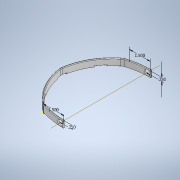
# Autodesk Inventor part: FaceMask_Part1
Saved by Autodesk Inventor 2020 (Build 240168000, 168)
## iProperties
Created: 2020-04-12
Part Number: FaceMask_Part1
Material: Generic
Document SubType Name: Modeling
Designer: maple
Density: 1 g/cm^3
Appearance: Default
Author: maple
Autodesk Inventor part; units mm, degrees
ref_plane "YZ Plane" through (0, 0, 0) normal (1, 0, 0) x (0, 1, 0)
sketch "Sketch1" plane through (0, 0, 0) normal (0, 1, 0) x (-1, 0, 0)
  line L0 (0, 0) -> (-76.2, 0)
  line L1 (-76.2, 0) -> (-76.2, -147.32)
  line L2 (-76.2, -147.32) -> (0, -147.32)
  line L3 (0, -147.32) -> (0, 0)
  line L4 (0, -73.66) -> (0, -139.7)
  line L5 (0, -73.66) -> (0, -7.62)
  line L6 (0, -73.66) -> (2.54, -73.66)
  line L7 (0, -40.64) -> (1.524, -40.64)
  line L8 (0, -106.68) -> (1.524, -106.68)
  arc A0 (2.54, -73.66) -> (0, -7.62) centre (-2148.078, -123.3072) ccw
  arc A1 (0, -139.7) -> (2.54, -73.66) centre (-2148.078, -24.0128) ccw
  arc A2 (-76.2, -147.32) -> (0, -139.7) centre (-57.15, 46.99) ccw
  arc A3 (0, -7.62) -> (-76.2, 0) centre (-57.15, -194.31) ccw
  line L9 (-76.2, 0) -> (-76.2, 2.54)
  line L10 (-37.7227, -0.0374) -> (-37.7227, 2.5026)
  line L11 (0, -7.62) -> (0, -5.08)
  line L12 (0, -139.7) -> (0, -142.24)
  line L13 (0, -139.7) -> (2.54, -139.7) construction
  line L14 (-37.7227, -147.2826) -> (-37.7227, -149.8226)
  line L15 (-76.2, -147.32) -> (-76.2, -149.86)
  arc A4 (0, -5.08) -> (-76.2, 2.54) centre (-57.15, -191.77) ccw
  arc A5 (-76.2, -149.86) -> (0, -142.24) centre (-57.15, 44.45) ccw
  line L16 (2.54, -73.66) -> (5.08, -73.66)
  line L17 (1.524, -40.64) -> (4.064, -40.64)
  line L18 (1.524, -106.68) -> (4.064, -106.68)
  arc A6 (5.08, -73.66) -> (0, -5.08) centre (-409.4814, -69.8901) ccw
  arc A7 (0, -142.24) -> (5.08, -73.66) centre (-409.4814, -77.4299) ccw
  line L19 (5.08, -73.66) -> (25.4, -73.66)
  line L20 (0, -40.64) -> (14.3684, -26.2716)
  line L21 (0, -40.64) -> (20.32, -40.64) construction
  line L22 (0, -106.68) -> (20.32, -106.68) construction
  arc A8 (25.4, -73.66) -> (0, -5.08) centre (-76.4718, -72.3966) ccw
  arc A9 (0, -142.24) -> (25.4, -73.66) centre (-76.4718, -74.9234) ccw
  line L23 (25.4, -73.66) -> (22.86, -73.66)
  line L24 (14.3684, -26.2716) -> (12.5724, -28.0676)
  line L25 (14.3684, -121.0484) -> (12.5724, -119.2524)
  arc A10 (22.86, -73.66) -> (0, -7.62) centre (-85.1784, -74.0814) ccw
  arc A11 (0, -139.7) -> (22.86, -73.66) centre (-85.1784, -73.2386) ccw
  line L26 (-76.2, -73.66) -> (-76.2, 7.62)
  line L27 (-76.2, -73.66) -> (-76.2, -154.94)
  line L28 (0, -73.66) -> (42.672, -73.66)
  line L29 (0, -5.08) -> (0, 0)
  line L30 (0, -142.24) -> (0, -147.32)
  line L31 (-76.2, 7.62) -> (-76.2, 5.08)
  line L32 (-37.7227, 7.5826) -> (-37.7227, 5.0426)
  line L33 (0, -147.32) -> (0, -147.32)
  line L34 (-76.2, -154.94) -> (-76.2, -152.4)
  line L35 (0, 0) -> (0, -2.54)
  line L36 (0, -147.32) -> (0, -144.78)
  line L37 (42.672, -73.66) -> (40.132, -73.66)
  line L38 (0, 0) -> (0, -40.64)
  line L39 (14.3684, -26.2716) -> (17.9605, -22.6795)
  line L40 (17.9605, -22.6795) -> (19.7566, -20.8834)
  line L41 (-37.7227, -149.8226) -> (-44.0727, -149.8226)
  line L42 (-44.0727, -149.8226) -> (-44.0727, -151.7279)
  line L43 (-44.0727, -151.7279) -> (-44.0727, -154.2679)
  line L44 (-20.4956, -147.32) -> (-20.4956, -149.86)
  line L45 (-20.4956, -149.86) -> (-20.4956, -152.4)
  arc A12 (-44.0727, -154.2679) -> (0, -147.32) centre (-43.0417, -17.5507) ccw
  arc A13 (-44.0727, -151.7279) -> (0, -144.78) centre (-43.0417, -15.0107) ccw
  line L46 (42.672, -73.66) -> (0, -147.32)
  line L47 (42.672, -73.66) -> (42.672, -148.1182)
  line L48 (42.672, -148.1182) -> (21.1194, -126.5656)
  line L49 (42.672, -148.1182) -> (73.152, -148.1182) construction
  arc A14 (0, -147.32) -> (42.672, -73.66) centre (-64.0407, -61.0304) ccw
  line L50 (21.1194, -126.5656) -> (19.3233, -124.7696)
  arc A15 (0, -144.78) -> (40.132, -73.66) centre (-68.6332, -59.1683) ccw
  line L51 (0, -147.32) -> (-38.1, -147.32)
  point P0 (0.4895, -8.2521)
  point P1 (0.4895, -139.0679)
  dimension "d0" = 76.2
  dimension "d1" = 147.32
  dimension "d2" = 66.04
  dimension "d3" = 66.04
  dimension "d4" = 2.54
  dimension "d5" = 1.524
  dimension "d6" = 1.524
  dimension "d7" = 2.54
  dimension "d8" = 2.54
  dimension "d9" = 2.54
  dimension "d10" = 2.54
  dimension "d11" = 90
  dimension "d12" = 2.54
  dimension "d13" = 2.54
  dimension "d14" = 2.54
  dimension "d15" = 2.54
  dimension "d16" = 2.54
  dimension "d17" = 20.32
  dimension "d18" = 20.32
  dimension "d19" = 45
  dimension "d20" = 20.32
  dimension "d22" = 2.54
  dimension "d23" = 2.54
  dimension "d24" = 2.54
  dimension "d34" = 81.28
  dimension "d35" = 81.28
  dimension "d36" = 42.672
  dimension "d37" = 5.08
  dimension "d38" = 5.08
  dimension "d39" = 5.08
  dimension "d41" = 2.54
  dimension "d42" = 2.54
  dimension "d46" = 2.54
  dimension "d47" = 2.54
  dimension "d48" = 2.54
  dimension "d49" = 2.54
  dimension "d50" = 40.64
  dimension "d51" = 5.08
  dimension "d52" = 2.54
  dimension "d55" = 6.35
  dimension "d56" = 2.54
  dimension "d57" = 2.54
  dimension "d58" = 2.54
  dimension "d59" = 30.48
  dimension "d60" = 135
  dimension "d61" = 2.54
  constraints: 104 end point, 50 point on circle, 16 centre point, 14 point on line, 12 horizontal, 9 vertical, 7 midpoint, 3 collinear, 3 equal length, 3 perpendicular, 2 parallel
  measures "d0" distance of L2.end L1.end
  measures "d1" distance of L1.end L0.end
  measures "d2" distance of L4.start L4.end
  measures "d3" distance of L4.start L5.end
  measures "d4" distance of L4.start L6.end
  measures "d5" distance of L7.start L7.end
  measures "d6" distance of L8.start L8.end
  measures "d7" distance of L0.end L9.end
  measures "d8" distance of L10.start L10.end
  measures "d9" distance of L5.end L11.end
  measures "d10" distance of L4.end L12.end
  measures "d11" angle of L12 L13
  measures "d12" distance of L14.start L14.end
  measures "d13" distance of L1.end L15.end
  measures "d14" distance of L6.end L16.end
  measures "d15" distance of L7.end L17.end
  measures "d16" distance of L8.end L18.end
  measures "d17" distance of L16.end L19.end
  measures "d18" distance of L7.start L20.end
  measures "d19" angle of L21 L20
  measures "d20" distance of L8.start L25.start
  measures "d22" distance of L19.end L23.end
  measures "d23" distance of L20.end L24.end
  measures "d24" distance of L25.start L25.end
  measures "d34" distance of L26.start L26.end
  measures "d35" distance of L26.start L27.end
  measures "d36" distance of L4.start L28.end
  measures "d37" distance of L11.end L29.end
  measures "d38" distance of L12.end L30.end
  measures "d39" distance of L10.end L32.start
  measures "d41" distance of L26.end L31.end
  measures "d42" distance of L32.start L32.end
  measures "d46" distance of L27.end L34.end
  measures "d47" distance of L29.end L35.end
  measures "d48" distance of L30.end L36.end
  measures "d49" distance of L28.end L37.end
  measures "d50" distance of L29.end L7.start
  measures "d51" distance of L20.end L39.end
  measures "d52" distance of L39.end L40.end
  measures "d55" distance of L14.end L41.end
  measures "d56" distance of L42.end L43.end
  measures "d57" distance of L44.start L44.end
  measures "d58" distance of L44.end L45.end
  measures "d59" distance of L47.end L48.end
  measures "d60" angle of L49 L48
  measures "d61" distance of L48.end L50.end
extrude "Extrusion2" add sketch "Sketch1" along normal blind 12.7 contours L28 L46 A15 | A14 L50 A15 L46 | A15 L46 L3 | L3 L2 A13 | A14 L46 A15 L50 | A12 L45 A13 L2 | L45 A12 L43 A13
ref_plane "Work Plane2" through (0, 0, -157.1625) normal (0, 0, 1) x (1, 0, 0)
sketch "Sketch2" plane through (0, 0, -157.1625) normal (0, 0, 1) x (1, 0, 0)
  line L0 (44.0727, 0) -> (0, 0) projected
  line L1 (0, 0) -> (38.1, 0)
  line L2 (38.1, 0) -> (38.1, 6.35)
  circle A0 centre (38.1, 6.35) radius 5.08
  dimension "d68" = 38.1
  dimension "d69" = 6.35
  dimension "d70" = 10.16
  constraints: 4 end point, 1 centre point, 1 coincident, 1 point on line, 1 vertical
  measures "d68" distance of L0.end L1.end
  measures "d69" distance of L1.end L2.end
  measures "d70" diameter of A0
extrude "Extrusion3" cut sketch "Sketch2" along normal blind 12.7
sketch "Sketch3" plane through (0, 0, 0) normal (0, 1, 0) x (-1, 0, 0)
  line L0 (42.672, -73.66) -> (40.132, -73.66) projected
  line L1 (42.672, -73.66) -> (0, -73.66)
  arc A0 (0, -147.32) -> (42.672, -73.66) centre (-64.0407, -61.0304) ccw projected
  line L2 (42.672, -73.66) -> (37.1128, -73.66)
  line L3 (37.1128, -73.66) -> (37.1128, -81.28)
  line L4 (37.1128, -81.28) -> (42.672, -81.28)
  line L5 (42.672, -81.28) -> (42.672, -73.66)
  line L6 (0, -73.66) -> (0, -93.8784)
  line L7 (0, -93.8784) -> (28.9412, -122.8196)
  line L8 (28.9412, -122.8196) -> (18.1649, -133.5959)
  line L9 (18.1649, -133.5959) -> (0, -115.431)
  line L10 (11.7489, -127.18) -> (22.5252, -116.4036)
  point P0 (0, 0)
  point P1 (16.6102, -132.0412)
  point P2 (25.9217, -119.8001)
  dimension "d73" = 7.62
  dimension "d74" = 20.2184
  dimension "d75" = 135
  dimension "d76" = 15.24
  constraints: 20 end point, 4 perpendicular, 3 point on line, 2 horizontal, 2 parallel, 1 vertical
  measures "d73" distance of L3.end L2.end
  measures "d74" distance of L1.end L6.end
  measures "d75" angle of L7 L6
  measures "d76" distance of L7.end L8.end
extrude "Extrusion4" cut sketch "Sketch3" along normal blind 1.905 contours A0 L4 L3 L1 L0 | L5 L4 A0 | A0 L9 L10 L7
ref_plane "Work Plane1" through (-42.672, 6.35, -73.66) normal (0, 0, 1) x (1, 0, 0)
mirror "Mirror2" about plane through (-42.672, 6.35, -73.66) normal (0, 0, 1) of "Extrusion2", "Extrusion3", "Extrusion4"
fillet "Fillet11" radius 12.7 6 edges at (0, 6.35, -2.54) (0, 6.35, -144.78) (0, 6.35, -147.32) (0, 6.35, 0) (-42.672, 7.3025, -73.66) (-40.132, 7.3025, -73.66)
fillet "Fillet12" radius 1.016 27 edges at (-42.5713, 12.7, -73.66) (-29.0892, 12.7, -32.6806) (22.8709, 12.7, 5.4557) (0.0698, 12.7, -147.1511) (22.8709, 12.7, -152.7757) (-29.0892, 12.7, -114.6394) (0.0947, 12.7, -144.5723) (23.0045, 12.7, -150.2556) (-27.0886, 12.7, -34.512) (23.0045, 12.7, 2.9356) (-27.0886, 12.7, -112.808) (0.0947, 0, -144.5723) (-8.7056, 0, -137.0052) (23.0045, 0, -150.2556) (0.0947, 0, -2.7477) (-8.7056, 0, -10.3148) (23.0045, 0, 2.9356) (0.0698, 0, -0.1689) (-9.5489, 0, -7.9846) (22.8709, 0, 5.4557) (-35.5861, 0, -46.0203) (-33.1039, 0, -47.049) (-33.1039, 0, -100.271) (-35.5861, 0, -101.2997) (0.0698, 0, -147.1511) (22.8709, 0, -152.7757) (-9.5489, 0, -139.3354)
fillet "Fillet13" radius 1.016 16 edges at (44.0727, 12.4024, -153.9703) (44.0727, 12.7, -152.9979) (44.0727, 12.4024, -152.0255) (44.0727, 6.35, -151.7279) (44.0727, 0.2976, -152.0255) (44.0727, 0, -152.9979) (44.0727, 0.2976, -153.9703) (44.0727, 6.35, -154.2679) (44.0727, 0, 5.6779) (44.0727, 0.2976, 6.6503) (44.0727, 6.35, 6.9479) (44.0727, 12.4041, 6.6487) (44.0727, 12.7, 5.6779) (44.0727, 12.4041, 4.7072) (44.0727, 6.35, 4.4079) (44.0727, 0.2976, 4.7055)
fillet "Fillet14" radius 0.762 38 edges at (-21.4852, 1.905, -126.0875) (-19.6848, 1.905, -124.2822) (-16.6102, 1.4605, -132.0412) (-15.7522, 0, -131.1832) (-15.1047, 0.2973, -130.5357) (-14.8934, 1.4605, -130.3244) (-16.3988, 0.2968, -131.8298) (-24.9817, 0, -118.8601) (-24.2572, 0.2954, -118.1356) (-24.0399, 1.4605, -117.9183) (-25.9217, 1.4605, -119.8001) (-25.7052, 0.2956, -119.5836) (-41.4916, 1.4605, -81.28) (-40.168, 0, -81.28) (-39.1479, 0.2957, -81.28) (-38.8422, 1.4605, -81.28) (-41.1868, 0.2959, -81.28) (-42.5713, 1.905, -73.66) (-42.0162, 1.905, -78.3231) (-40.0048, 1.905, -73.66) (-39.3902, 1.905, -78.4252) (-40.168, 0, -66.04) (-39.1479, 0.2957, -66.04) (-38.8422, 1.4605, -66.04) (-41.4916, 1.4605, -66.04) (-41.1868, 0.2959, -66.04) (-15.7522, 0, -16.1368) (-15.1047, 0.2973, -16.7843) (-14.8934, 1.4605, -16.9956) (-16.6102, 1.4605, -15.2788) (-16.3988, 0.2968, -15.4902) (-25.9217, 1.4605, -27.5199) (-24.9817, 0, -28.4599) (-24.2572, 0.2954, -29.1844) (-24.0399, 1.4605, -29.4017) (-25.7052, 0.2956, -27.7364) (-21.4852, 1.905, -21.2325) (-19.6848, 1.905, -23.0378)
sketch "Sketch4" plane through (0, 0, -157.1625) normal (0, 0, 1) x (1, 0, 0)
  line L0 (0, 0) -> (38.1, 0)
  line L1 (-2.6391, 0) -> (2.1126, 0) projected
  line L2 (38.1, 0) -> (38.1, 6.35)
  dimension "d83" = 38.1
  dimension "d84" = 6.35
  constraints: 4 end point, 1 coincident, 1 collinear, 1 perpendicular
  measures "d83" distance of L0.start L0.end
  measures "d84" distance of L0.end L2.end
sketch "Sketch5" plane through (0, 0, 0) normal (0, 0, 1) x (1, 0, 0)
  line L0 (0, 0) -> (38.1, 0)
  line L1 (-2.6391, 0) -> (2.1126, 0) projected
  line L2 (38.1, 0) -> (38.1, 6.35)
  dimension "d85" = 38.1
  dimension "d86" = 6.35
  constraints: 4 end point, 1 collinear, 1 perpendicular
  measures "d85" distance of L0.start L0.end
  measures "d86" distance of L0.end L2.end
body "Solid2"
